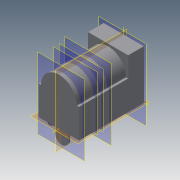
# Autodesk Inventor part: MJ179PH
Saved by Autodesk Inventor 2015 SP1 (Build 190203100, 203)
## iProperties
Created: 2015-03-31
Part Number: MJ179PH
Material: 一般
Document SubType Name: Modeling
Designer: Yamaura
Density: 1 g/cm^3
Appearance: 既定
Author: Yamaura
Autodesk Inventor part; units mm, degrees
sketch "スケッチ1" plane through (0, 0, 0) normal (0, 1, 0) x (-1, 0, 0)
  line L0 (-4.5, 11) -> (4.5, 11)
  line L1 (4.5, 11) -> (4.5, 0)
  line L2 (4.5, 0) -> (-4.5, 0)
  line L3 (-4.5, 0) -> (-4.5, 11)
  point P0 (0, 0)
  dimension "d0" = 9
  dimension "d1" = 4.5
  dimension "d2" = 11
  constraints: 8 end point, 2 parallel, 1 horizontal, 1 midpoint, 1 perpendicular
  measures "d0" distance of L0.start L0.end
  measures "d1" distance from line of L3 point (0, 0)
  measures "d2" distance of L0.end L1.end
extrude "押し出し1" add sketch "スケッチ1" against normal blind 3.5
sketch "スケッチ3" plane through (0, 0, 0) normal (0, 1, 0) x (-1, 0, 0)
  circle A0 centre (0, 6.5) radius 4
  line L0 (-4, 6.5) -> (4, 6.5)
  line L1 (4, 6.5) -> (4, 0)
  line L2 (4, 0) -> (-4, 0)
  line L3 (-4, 0) -> (-4, 6.5)
  point P0 (0, 0)
  dimension "d9" = 8
  dimension "d10" = 6.5
  constraints: 8 end point, 2 parallel, 1 horizontal, 1 horizontal alignment, 1 perpendicular, 2 other
  measures "d10" distance of point (0, 6.5) point (0, 0)
extrude "押し出し3" add sketch "スケッチ3" against normal blind 14.5
ref_plane "作業平面1" through (0, -9.5, 0) normal (0, 1, 0) x (-1, 0, 0)
sketch "スケッチ4" plane through (0, 0, 0) normal (0, 1, 0) x (-1, 0, 0)
  point P0 (0, 0)
sketch "スケッチ5" plane through (0, 0, 0) normal (0, 1, 0) x (-1, 0, 0)
  line L0 (-4.5, 0) -> (4.5, 0)
  line L1 (4.5, 0) -> (4.5, 6.5)
  line L2 (4.5, 6.5) -> (-4.5, 6.5)
  line L3 (-4.5, 6.5) -> (-4.5, 0)
  point P0 (0, 0)
  dimension "d14" = 4.5
  dimension "d15" = 9
  dimension "d16" = 6.5
  constraints: 8 end point, 2 parallel, 1 horizontal, 1 perpendicular
  measures "d14" distance from line of L3 point (0, 0)
  measures "d15" distance of L0.start L0.end
  measures "d16" distance of L0.end L1.end
extrude "押し出し4" add sketch "スケッチ5" against normal blind 14.5
sketch "スケッチ6" plane through (0, -9.5, 0) normal (0, 1, 0) x (-1, 0, 0)
  line L0 (5.1, 5) -> (4.9, 5)
  line L1 (4.9, 5) -> (4.9, -3.5)
  line L2 (4.9, -3.5) -> (5.1, -3.5)
  line L3 (5.1, -3.5) -> (5.1, 5)
  line L4 (0, -13.24) -> (0, 15.04) projected
  line L5 (4.7, 5) -> (4.9, 5)
  line L6 (4.9, 5) -> (4.9, -3.5)
  line L7 (4.9, -3.5) -> (4.7, -3.5)
  line L8 (4.7, -3.5) -> (4.7, 5)
  line L9 (5.1, 5) -> (0, 5)
  line L10 (0, 5) -> (0, 4.6)
  line L11 (0, 4.6) -> (5.1, 4.6)
  line L12 (5.1, 4.6) -> (5.1, 5)
  point P0 (0, 0)
  dimension "d19" = 4.9
  dimension "d20" = 0.2
  dimension "d21" = 3.5
  dimension "d22" = 5
  dimension "d27" = 0.2
  dimension "d28" = 0.4
  constraints: 24 end point, 6 parallel, 3 horizontal, 3 perpendicular, 1 point on line
  measures "d19" distance between parallel lines of L4 L1
  measures "d20" distance of L1.end L2.end
  measures "d21" distance from line of L2 point (0, 0)
  measures "d22" distance from line of L0 point (0, 0)
  measures "d27" distance of L1.end L7.end
  measures "d28" distance of L10.end L9.end
extrude "押し出し5" add sketch "スケッチ6" against normal blind 2.5
ref_plane "作業平面2" through (0, -10.75, 0) normal (0, 1, 0) x (-1, 0, 0)
fillet "フィレット1" radius 0.4 1 edges at (-5.1, -10.75, 5)
ref_plane "作業平面4" through (0, -13.7, 0) normal (0, 1, 0) x (-1, 0, 0)
sketch "スケッチ7" plane through (0, -13.7, 0) normal (0, 1, 0) x (-1, 0, 0)
  line L0 (1.5, 5.7) -> (-1.5, 5.7)
  line L1 (-1.5, 5.7) -> (-1.5, -3.4)
  line L2 (-1.5, -3.4) -> (1.5, -3.4)
  line L3 (1.5, -3.4) -> (1.5, 5.7)
  point P0 (0, 0)
  dimension "d31" = 1.5
  dimension "d32" = 3
  constraints: 8 end point, 2 parallel, 1 horizontal, 1 perpendicular
  measures "d31" distance from line of L3 point (0, 0)
  measures "d32" distance of L1.end L2.end
extrude "押し出し6" add sketch "スケッチ7" along normal mid plane 0.4
fillet "フィレット2" radius 1.5 1 edges at (-1.5, -13.7, -3.4)
fillet "フィレット2" radius 1.5 1 edges at (1.5, -13.7, -3.4)
ref_plane "作業平面5" through (0, -7.7, 0) normal (0, 1, 0) x (-1, 0, 0)
sketch "スケッチ8" plane through (0, -7.7, 0) normal (0, 1, 0) x (-1, 0, 0)
  line L0 (1.25, 6.5) -> (-1.25, 6.5)
  line L1 (-1.25, 6.5) -> (-1.25, -3.5)
  line L2 (-1.25, -3.5) -> (1.25, -3.5)
  line L3 (1.25, -3.5) -> (1.25, 6.5)
  line L4 (4.5, 0) -> (-4.5, 0) projected
  point P0 (0, 0)
  dimension "d38" = 3.5
  dimension "d39" = 2.5
  dimension "d40" = 1.25
  dimension "d41" = 6.5
  constraints: 8 end point, 2 parallel, 1 horizontal, 1 perpendicular
  measures "d38" distance between parallel lines of L2 L4
  measures "d39" distance of L1.end L2.end
  measures "d40" distance from line of L3 point (0, 0)
  measures "d41" distance from line of L0 point (0, 0)
extrude "押し出し7" add sketch "スケッチ8" along normal mid plane 0.4
fillet "フィレット3" radius 1.25 1 edges at (1.25, -7.7, -3.5)
fillet "フィレット3" radius 1.25 3 edges at (-1.25, -7.7, -3.5) (-4.9, -9.5, -3.5) (-4.9, -12, -3.5)
sketch "スケッチ9" plane through (0, 0, 0) normal (0, 1, 0) x (-1, 0, 0)
  circle A0 centre (0, 6.5) radius 3
  point P0 (0, 0)
  dimension "d46" = 6
  dimension "d47" = 6.5
  constraints: 1 centre point
  measures "d46" diameter of A0
  measures "d47" distance of A0.centre point (0, 0)
extrude "押し出し8" cut sketch "スケッチ9" against normal blind 10
sketch "スケッチ2" plane through (0, 0, 0) normal (0, 1, 0) x (-1, 0, 0)
  circle A0 centre (0, 6.5) radius 3
  line L0 (4.5, 0) -> (-4.5, 0) projected
  point P0 (0, 0)
  dimension "d5" = 6
  dimension "d6" = 6.5
  constraints: 1 centre point
  measures "d5" diameter of A0
  measures "d6" distance from line of A0.centre L0
